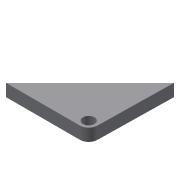
# Autodesk Inventor part: 00_penholder_servomotor
Saved by Autodesk Inventor 2019.4 (Build 234330000, 330)
## iProperties
Created: 2021-10-05
Part Number: 00_penholder_servomotor
Material: Generic
Document SubType Name: Modeling
Designer: diederichbenedict
Density: 1 g/cm^3
Appearance: Default
Author: diederichbenedict
Autodesk Inventor part; units mm, degrees
ref_plane "YZ Plane" through (0, 0, 0) normal (1, 0, 0) x (0, 1, 0)
ref_plane "XZ Plane" through (0, 0, 0) normal (0, 1, 0) x (-1, 0, 0)
ref_plane "XY Plane" through (0, 0, 0) normal (0, 0, 1) x (1, 0, 0)
sketch "Sketch1" plane through (0, 0, 0) normal (0, 1, 0) x (-1, 0, 0)
  circle A0 centre (0, 0) radius 2.35
  circle A1 centre (0, 0) radius 3.5
  dimension "d0" = 4.7
  dimension "d1" = 7
  constraints: 2 centre point, 2 coincident
  measures "d0" diameter of A0
  measures "d1" diameter of A1
extrude "Extrusion1" add sketch "Sketch1" along normal blind 7
sketch "Sketch2" plane through (0, 7, 0) normal (0, 1, 0) x (1, 0, 0)
  circle A0 centre (0, 0) radius 2.35 projected
  circle A1 centre (0, 0) radius 3.5 projected
  line L0 (0, -3.5) -> (-30, -3.5)
  line L1 (-30, -3.5) -> (4.0254, 30.5254)
  line L2 (4.0254, 30.5254) -> (3.4995, -0.0602)
  circle A2 centre (0, 0) radius 3.5 projected
  dimension "d4" = 30
  dimension "d5" = 45
  constraints: 6 end point, 1 horizontal, 1 point on circle, 1 tangent, 1 vertical alignment, 1 other
  measures "d4" distance of L0.start L0.end
  measures "d5" angle of L0 L1
extrude "Extrusion2" add sketch "Sketch2" against normal up to surface (7 mm away) contours A1 L0 L1 L2
ref_plane "Work Plane1" through (3.4403, 0, 3.5) normal (0.7131596, 0, -0.7010017) x (0, 1, 0)
sketch "Sketch3" plane through (3.4403, 0, 3.5) normal (0.7131596, 0, -0.7010017) x (0, 1, 0)
  line L0 (7, -23.8554) -> (0, -23.8554) projected
  circle A0 centre (3.5, -30.2668) radius 7.3045
  line L1 (0, -23.8554) -> (0, -2.4117) projected
  line L2 (7, -2.4117) -> (7, -23.8554) projected
  point P0 (0, -4.9077)
  dimension "d18" = 7
  dimension "d19" = 3.5
  constraints: 3 other
  measures "d18" distance between parallel lines of L1 L2
  measures "d19" distance from line of point (3.5, -30.267) L2
extrude "Extrusion3" cut sketch "Sketch3" along normal through all both and the other way through all
sketch "Sketch4" plane through (0, 0, 0) normal (0, -1, 0) x (1, 0, 0)
  line L0 (-0.0168, -23.4826) -> (-4.2595, -19.24)
  line L1 (-4.2595, -19.24) -> (-3.0174, -17.9979)
  line L2 (-3.0174, -17.9979) -> (1.2253, -22.2405)
  line L3 (1.2253, -22.2405) -> (-0.0168, -23.4826)
  line L4 (-0.0168, -23.4826) -> (-3.0174, -17.9979) construction
  line L5 (-4.2595, -19.24) -> (1.2253, -22.2405) construction
  line L6 (-30, 3.5) -> (4.0254, -30.5254) projected
  line L7 (-22.7408, -0.9308) -> (-18.4981, -5.1734)
  line L8 (-18.4981, -5.1734) -> (-17.0839, -3.7592)
  line L9 (-17.0839, -3.7592) -> (-21.3266, 0.4834)
  line L10 (-21.3266, 0.4834) -> (-22.7408, -0.9308)
  line L11 (-22.7408, -0.9308) -> (-17.0839, -3.7592) construction
  line L12 (-18.4981, -5.1734) -> (-21.3266, 0.4834) construction
  point P0 (0, 0)
  point P1 (-1.5171, -20.7403)
  point P2 (-19.9124, -2.345)
  dimension "d10" = 3
  dimension "d11" = 6
  dimension "d12" = 6
  dimension "d13" = 2
  dimension "d14" = 2
  constraints: 24 end point, 6 parallel, 4 midpoint, 2 perpendicular
  measures "d10" distance from line of L6 point (-1.517, -20.74)
  measures "d11" distance between parallel lines of L1 L3
  measures "d12" distance of L7.start L7.end
  measures "d13" distance of L8.end L7.end
  measures "d14" distance between parallel lines of L7 L6
extrude "Extrusion4" cut sketch "Sketch4" against normal through all
fillet "Fillet1" radius 2 2 edges at (4.0035, 3.5, -29.2516) (-29.3161, 3.5, 3.5)
equation "\"d19\" = 0.5 * d18"
body "Solid1"
